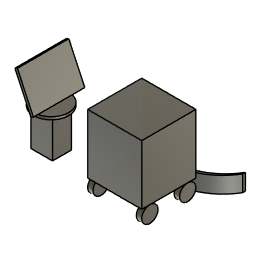
Prototype v1 (Autodesk Fusion 360 design; units mm, degrees)
Autodesk Fusion 360 part; units mm, degrees
sketch "Esquisse1" plane through (0, 0, 0) normal (0, 0, 1) x (1, 0, 0)
  line L0 (0.5, 0.5) -> (2.5, 0.5)
  line L1 (2.5, 0.5) -> (2.5, 2.5)
  line L2 (2.5, 2.5) -> (0.5, 2.5)
  line L3 (0.5, 2.5) -> (0.5, 0.5)
  constraint horizontal L0
  constraint vertical L1
  constraint horizontal L2
  constraint vertical L3
extrude "Extrusion1" add sketch "Esquisse1" along normal blind 2.2 makes body 1
sketch "Esquisse2" plane through (2.5, 0, 0) normal (1, 0, 0) x (0, 1, 0)
  line L0 (0.5, 0) -> (2.5, 0)
  line L1 (2.5, 0) -> (2.5, 2.2)
  line L2 (2.5, 2.2) -> (0.5, 2.2)
  line L3 (0.5, 2.2) -> (0.5, 0)
  circle A0 centre (0.8, -0.3) radius 0.3
  circle A1 centre (0.8, -0.3) radius 0.3
  circle A2 centre (2.2, -0.3) radius 0.3
  point P0 (0.8, -0.3)
  point P1 (0.8, -0.3)
  point P2 (2.2, -0.3)
  constraint tangent L0 A0
extrude "Extrusion2" add sketch "Esquisse2" against normal blind 0.2 separate body contours A2 | A0 A1 picked at (2.270059, -0.232719) picked at (1.022161, -0.367372) makes body 2 at (2.366667, 1.098509, -0.32987) makes body 3 at (2.366667, 2.498509, -0.32987)
sketch "Esquisse3" plane through (0.5, 0, 0) normal (-1, 0, 0) x (0, -1, 0)
  line L0 (-2.5, 0) -> (-0.5, 0)
  line L1 (-0.5, 0) -> (-0.5, 2.2)
  line L2 (-0.5, 2.2) -> (-2.5, 2.2)
  line L3 (-2.5, 2.2) -> (-2.5, 0)
  circle A0 centre (-2.2, -0.3) radius 0.3
  circle A1 centre (-0.8, -0.3) radius 0.3
  constraint tangent L0 A0
  constraint tangent L0 A1
extrude "Extrusion3" add sketch "Esquisse3" against normal blind 0.2 separate body contours A1 | A0 picked at (-0.902824, -0.313593) picked at (-2.329049, -0.284654) makes body 4 at (0.633333, 1.901491, -0.32987) makes body 5 at (0.633333, 0.501491, -0.32987)
sketch "Esquisse4" plane through (0, 0, 0) normal (0, 0, -1) x (1, 0, 0)
  line L0 (0.5, -0.5) -> (0.5, -2.5)
  line L1 (0.5, -2.5) -> (2.5, -2.5)
  line L2 (2.5, -2.5) -> (2.5, -0.5)
  line L3 (2.5, -0.5) -> (0.5, -0.5)
  arc A0 (3.232051, -3.5) -> (-0.232051, -3.5) centre (1.5, -4.5) ccw
  arc A1 (3.232051, -3.5) -> (-0.232051, -3.5) centre (1.5, -4.5) ccw
  arc A2 (3.232051, -3.6) -> (-0.232051, -3.6) centre (1.5, -4.6) ccw
  line L4 (-0.232051, -3.6) -> (-0.232051, -3.5)
  line L5 (3.232051, -3.6) -> (3.232051, -3.5)
  constraint tangent L1 A0
  constraint vertical L4
  constraint parallel L4 L5
extrude "Extrusion4" add sketch "Esquisse4" against normal blind 0.4 separate body contours A0 A1 A2 L4 L5 picked at (1.599361, -2.540779) makes body 6
move_body "Déplacer1" bodies 6 to x (1, 0, 0) y (0, 1, 0) z (0, 0, 1) at (0, 0, -0.6)
extrude "Extrusion5" add 1 faces at (1.599361, 2.540779, -0.2) along direction (0, 0, 1) blind 0.2 on bodies 6 bodies 6 2 3 4 5 1
sketch "Esquisse5" plane through (0, 2.5, 0) normal (0, 1, 0) x (-1, 0, 0)
  line L0 (-2.5, 0) -> (-1.5, 0)
  line L1 (-1.5, 0) -> (-0.5, 0)
  line L2 (-0.5, 0) -> (-0.5, 2.2)
  line L3 (-0.5, 2.2) -> (-2.5, 2.2)
  line L4 (-2.5, 2.2) -> (-2.5, 0)
  line L5 (-1.9, 1.2) -> (-1.2, 1.2)
  line L6 (-1.2, 1.2) -> (-1.2, 0.8)
  line L7 (-1.2, 0.8) -> (-1.9, 0.8)
  line L8 (-1.9, 0.8) -> (-1.9, 1.2)
  constraint horizontal L5
  constraint vertical L6
  constraint horizontal L7
  constraint vertical L8
extrude "Extrusion6" add sketch "Esquisse5" along normal blind 0.2 separate body contours L5 L6 L7 L8 picked at (-1.666667, 1.066667) makes body 7
sketch "Esquisse6" plane through (0.5, 0, 0) normal (-1, 0, 0) x (0, -1, 0)
  line L0 (-2.5, 0) -> (-0.5, 0)
  line L1 (-0.5, 0) -> (-0.5, 2.2)
  line L2 (-0.5, 2.2) -> (-2.5, 2.2)
  line L3 (-2.5, 2.2) -> (-2.5, 0)
sketch "Esquisse7" plane through (0, 0, 0) normal (0, 0, 1) x (1, 0, 0)
  line L0 (-1.3, 1) -> (-2.1, 1)
  line L1 (-2.1, 1) -> (-2.1, 1.7)
  line L2 (-2.1, 1.7) -> (-1.3, 1.7)
  line L3 (-1.3, 1.7) -> (-1.3, 1)
  constraint horizontal L0
  constraint vertical L1
  constraint horizontal L2
  constraint vertical L3
extrude "Extrusion7" add sketch "Esquisse7" along normal blind 2.2 separate body makes body 8
sketch "Esquisse8" plane through (0, 0, 2.2) normal (0, 0, 1) x (-1, 0, 0)
  line L0 (1.3, -1.7) -> (2.1, -1.7)
  line L1 (2.1, -1.7) -> (2.1, -1)
  line L2 (2.1, -1) -> (1.3, -1)
  line L3 (1.3, -1) -> (1.3, -1.7)
  circle A0 centre (1.7, -1.35) radius 0.65
extrude "Extrusion8" add sketch "Esquisse8" along normal blind 0.1 contours L0 L1 L2 L3 | A0 picked at (1.566667, -1.233333) picked at (1.683808, -0.900606) bodies 8
sketch "Esquisse9" plane through (0, 0, 2.3) normal (0, 0, 1) x (-1, 0, 0)
  circle A0 centre (1.7, -1.35) radius 0.65
  line L0 (1.5, -1.1) -> (1.6, -1.1)
  line L1 (1.6, -1.1) -> (1.6, -1.8)
  line L2 (1.6, -1.8) -> (1.5, -1.8)
  line L3 (1.5, -1.8) -> (1.5, -1.1)
  constraint horizontal L0
  constraint vertical L1
  constraint horizontal L2
  constraint vertical L3
extrude "Extrusion9" add sketch "Esquisse9" along normal blind 1.1 contours L0 L1 L2 L3 picked at (1.533333, -1.333333) bodies 8
extrude "Extrusion10" add 1 faces at (-1.566667, 1.8, 2.666667) along direction (0, 1, 0) blind 0.6 on bodies 8 bodies 8
extrude "Extrusion11" add 1 faces at (-1.533333, 1.1, 2.666667) along direction (0, -1, 0) blind 0.6 on bodies 8 bodies 8
extrude "Extrusion12" add 1 faces at (-1.566667, 1.133333, 3.4) along direction (0, 0, 1) blind 0.3 on bodies 8 bodies 8
split "Scinder1" by plane through (-1.6, 1.8, 2.3) normal (0, 0, -1) bodies 8 makes body 9 at (-1.833333, 1.7, 0.733333)
move_body "Déplacer2" bodies 8 to x (0.90630779, 0, 0.42261826) y (0, 1, 0) z (-0.42261826, 0, 0.90630779) at (0.781097, 0.043224, 0.85338)
sketch "Esquisse10" plane through (0, 1, 0) normal (0, -1, 0) x (1, 0, 0)
  line L0 (-2.1, 0) -> (-1.3, 0)
  line L1 (-1.3, 0) -> (-1.3, 2.2)
  line L2 (-1.3, 2.2) -> (-2.1, 2.2)
  line L3 (-2.1, 2.2) -> (-2.1, 0)
  line L4 (-2.1, 0.8) -> (-1.3, 0.8)
  constraint coincident L1 L4.end
  constraint perpendicular L1 L4
split "Scinder2" by curves path "Esquisse10" along L4 bodies 9 makes body 10 at (-1.566667, 1, 0.266667)
delete_body "RemoveBody1" bodies 10
move_body "Déplacer3" bodies 9 8 to x (1, 0, 0) y (0, 1, 0) z (0, 0, 1) at (0, 0, -1.4)
sketch "Esquisse11" plane through (0.5, 0, 0) normal (-1, 0, 0) x (0, -1, 0)
  circle A0 centre (-1.7, 1.5) radius 0.090723
extrude "Extrusion13" cut sketch "Esquisse11" against normal blind 0.9 bodies 6
sketch "Esquisse12" plane through (0.5, 0, 0) normal (-1, 0, 0) x (0, -1, 0)
  circle A0 centre (-1.7, 1.5) radius 0.094152
extrude "Extrusion14" add sketch "Esquisse12" along normal blind 0.95 separate body makes body 11
copy_body "Corps->Comp1" bodies 11 removing the originals makes body 12 in component "Component"
component "Component" placed x (1, 0, 0) y (0, 1, 0) z (0, 0, 1) at (0.95, 0, 0)
